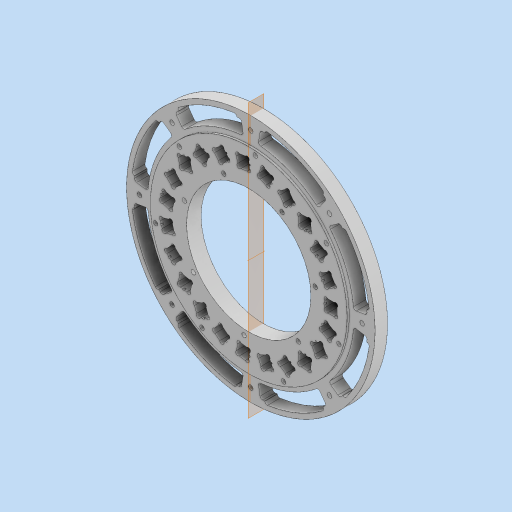
# Autodesk Inventor part: Ring_945
Saved by Autodesk Inventor 2024.2 (Build 282272000, 272)
## iProperties
Created: 2025-04-23
Part Number: Ring_945
Material: Generic
Document SubType Name: Modeling
Designer: 23661194
Density: 1 g/cm^3
Appearance: Default
Author: 23661194
Autodesk Inventor part; units mm, degrees
ref_plane "XZ Plane" through (0, 0, 0) normal (0, 1, 0) x (-1, 0, 0)
ref_plane "XY Plane" through (0, 0, 0) normal (0, 0, 1) x (1, 0, 0)
sketch "Shim Tray Slot_1" plane through (0, 0, 0) normal (0, 0, 1) x (1, 0, 0)
  line L0 (30.092, 109.0254) -> (29.9458, 108.3375)
  line L1 (33.5758, 105.3229) -> (31.6829, 97.1237)
  line L2 (-33.5758, 105.3229) -> (-31.6821, 97.1202)
  line L3 (-30.092, 109.0254) -> (-29.9458, 108.3375)
  arc A0 (-32.2001, 107.689) -> (-33.5758, 105.3229) centre (-31.6271, 105.7728) ccw
  arc A1 (29.147, 95.658) -> (-29.1504, 95.657) centre (0, 0) ccw
  arc A2 (28.6337, 111.3782) -> (-28.6337, 111.3782) centre (0, 0) ccw
  arc A3 (-29.9458, 108.3375) -> (-32.2001, 107.689) centre (0, 0) ccw
  arc A4 (32.2001, 107.689) -> (29.9458, 108.3375) centre (0, 0) ccw
  arc A5 (-28.6337, 111.3782) -> (-30.092, 109.0254) centre (-28.1357, 109.4412) ccw
  arc A6 (-31.6821, 97.1202) -> (-29.1504, 95.657) centre (-29.7334, 97.5701) ccw
  arc A7 (29.147, 95.658) -> (31.6829, 97.1237) centre (29.7309, 97.5743) ccw
  arc A8 (33.5758, 105.3229) -> (32.2001, 107.689) centre (31.6271, 105.7728) ccw
  arc A9 (30.092, 109.0254) -> (28.6337, 111.3782) centre (28.1357, 109.4412) ccw
  line L4 (0, 0) -> (0, 107.5)
  arc A10 (33.9656, 105.2329) -> (32.3146, 108.0722) centre (31.6271, 105.7728) ccw
  line L5 (33.9656, 105.2329) -> (32.0726, 97.0337)
  arc A11 (29.0304, 95.2754) -> (32.0726, 97.0337) centre (29.7309, 97.5743) ccw
  arc A12 (29.0304, 95.2754) -> (-29.0338, 95.2743) centre (0, 0) ccw
  arc A13 (-32.0718, 97.0302) -> (-29.0338, 95.2743) centre (-29.7334, 97.5701) ccw
  line L6 (-32.0718, 97.0302) -> (-33.9656, 105.2329)
  arc A14 (-32.3146, 108.0722) -> (-33.9656, 105.2329) centre (-31.6271, 105.7728) ccw
  arc A15 (-30.4152, 108.6221) -> (-32.3146, 108.0722) centre (0, 0) ccw
  line L7 (-30.4152, 108.6221) -> (-30.4833, 108.9422)
  arc A16 (-28.7333, 111.7656) -> (-30.4833, 108.9422) centre (-28.1357, 109.4412) ccw
  arc A17 (28.7333, 111.7656) -> (-28.7333, 111.7656) centre (0, 0) ccw
  arc A18 (30.4833, 108.9422) -> (28.7333, 111.7656) centre (28.1357, 109.4412) ccw
  line L8 (30.4833, 108.9422) -> (30.4152, 108.6221)
  arc A19 (32.3146, 108.0722) -> (30.4152, 108.6221) centre (0, 0) ccw
  dimension "d124" = 22.5
  dimension "d134" = 0.4
  measures "d134" radial gap between concentric circles of A2 A17
sketch "Shim Tray Slot_1_1" plane through (0, 0, 0) normal (0, 0, 1) x (1, 0, 0)
  line L0 (30.092, 109.0254) -> (29.9458, 108.3375)
  line L1 (33.5758, 105.3229) -> (31.6821, 97.1202)
  line L2 (-33.5758, 105.3229) -> (-31.6821, 97.1202)
  line L3 (-30.092, 109.0254) -> (-29.9458, 108.3375)
  arc A0 (-32.2001, 107.689) -> (-33.5758, 105.3229) centre (-31.6271, 105.7728) ccw
  arc A1 (29.1504, 95.657) -> (-29.1504, 95.657) centre (0, 0) ccw
  arc A2 (28.6337, 111.3782) -> (-28.6337, 111.3782) centre (0, 0) ccw
  arc A3 (-29.9458, 108.3375) -> (-32.2001, 107.689) centre (0, 0) ccw
  arc A4 (32.2001, 107.689) -> (29.9458, 108.3375) centre (0, 0) ccw
  arc A5 (-28.6337, 111.3782) -> (-30.092, 109.0254) centre (-28.1357, 109.4412) ccw
  arc A6 (-31.6821, 97.1202) -> (-29.1504, 95.657) centre (-29.7334, 97.5701) ccw
  arc A7 (29.1504, 95.657) -> (31.6821, 97.1202) centre (29.7309, 97.5743) ccw
  arc A8 (33.5758, 105.3229) -> (32.2001, 107.689) centre (31.6271, 105.7728) ccw
  arc A9 (30.092, 109.0254) -> (28.6337, 111.3782) centre (28.1357, 109.4412) ccw
  line L4 (0, 0) -> (0, 107.5)
  dimension "d125" = 22.5
  dimension "d126" = 22.5
sketch "Sketch1" plane through (0, 0, 0) normal (0, 0, 1) x (1, 0, 0)
  circle A0 centre (0, 0) radius 60
  circle A1 centre (0, 0) radius 120
  circle A2 centre (0, 0) radius 95
  dimension "d0" = 120
  dimension "d1" = 240
  dimension "d2" = 190
  constraints: 3 centre point, 3 coincident
  measures "d0" diameter of A0
  measures "d1" diameter of A1
  measures "d2" diameter of A2
extrude "Extrusion1" add sketch "Sketch1" along normal blind 12 contours A1 | A2
extrude "Extrusion2" add sketch "Sketch1" along normal blind 14 contours A2
sketch "Sketch3" plane through (0, 0, 14) normal (0, 0, 1) x (1, 0, 0)
  circle A0 centre (0, 0) radius 79.3546
  line L0 (79.3546, 0) -> (0, 0)
  line L1 (76.4119, 21.4096) -> (0, 0)
  line L2 (67.8021, 41.2314) -> (0, 0)
  line L3 (54.1637, 57.9952) -> (0, 0)
  line L4 (36.5083, 70.4577) -> (0, 0)
  line L5 (16.1452, 77.6948) -> (0, 0)
  line L6 (-5.4153, 79.1696) -> (0, 0)
  line L7 (-26.5742, 74.7727) -> (0, 0)
  line L8 (-45.7622, 64.8303) -> (0, 0)
  line L9 (-61.5562, 50.0797) -> (0, 0)
  line L10 (-72.7849, 31.6149) -> (0, 0)
  line L11 (-78.6155, 10.8054) -> (0, 0)
  line L12 (-78.6155, -10.8054) -> (0, 0)
  line L13 (-72.7849, -31.6149) -> (0, 0)
  line L14 (-61.5562, -50.0797) -> (0, 0)
  line L15 (-45.7622, -64.8303) -> (0, 0)
  line L16 (-26.5742, -74.7727) -> (0, 0)
  line L17 (-5.4153, -79.1696) -> (0, 0)
  line L18 (16.1452, -77.6948) -> (0, 0)
  line L19 (36.5083, -70.4577) -> (0, 0)
  line L20 (54.1637, -57.9952) -> (0, 0)
  line L21 (67.8021, -41.2314) -> (0, 0)
  line L22 (76.4119, -21.4096) -> (0, 0)
  line L23 (-168, 0) -> (168, 0) projected
  line L24 (85.2946, 5.94) -> (73.4146, 5.94)
  line L25 (73.4146, 5.94) -> (73.4146, -5.94)
  line L26 (73.4146, -5.94) -> (85.2946, -5.94)
  line L27 (85.2946, -5.94) -> (85.2946, 5.94)
  line L28 (85.2946, 5.94) -> (73.4146, -5.94) construction
  line L29 (73.4146, 5.94) -> (85.2946, -5.94) construction
  circle A1 centre (79.3546, 0) radius 2
  circle A2 centre (74.8276, -4.527) radius 2.1
  circle A3 centre (83.8816, -4.527) radius 2.1
  circle A4 centre (83.8816, 4.527) radius 2.1
  circle A5 centre (74.8276, 4.527) radius 2.1
  circle A6 centre (73.0546, 0) radius 0.75
  line L30 (73.0546, 0) -> (79.3546, 0)
  line L31 (78.4008, 29.5712) -> (68.2503, 23.3985)
  line L32 (68.2503, 23.3985) -> (74.423, 13.248)
  line L33 (74.423, 13.248) -> (84.5735, 19.4207)
  line L34 (84.5735, 19.4207) -> (78.4008, 29.5712)
  line L35 (78.4008, 29.5712) -> (74.423, 13.248) construction
  line L36 (68.2503, 23.3985) -> (84.5735, 19.4207) construction
  circle A7 centre (76.4119, 21.4096) radius 2
  circle A8 centre (74.8961, 15.1895) radius 2.1
  circle A9 centre (82.632, 19.8938) radius 2.1
  circle A10 centre (77.9277, 27.6297) radius 2.1
  circle A11 centre (70.1918, 22.9254) radius 2.1
  circle A12 centre (71.029, 18.1362) radius 0.75
  line L37 (71.029, 18.1362) -> (76.4119, 21.4096)
  line L38 (65.2608, 49.2382) -> (59.7953, 38.6901)
  line L39 (59.7953, 38.6901) -> (70.3433, 33.2245)
  line L40 (70.3433, 33.2245) -> (75.8089, 43.7726)
  line L41 (75.8089, 43.7726) -> (65.2608, 49.2382)
  line L42 (65.2608, 49.2382) -> (70.3433, 33.2245) construction
  line L43 (59.7953, 38.6901) -> (75.8089, 43.7726) construction
  circle A13 centre (67.8021, 41.2314) radius 2
  circle A14 centre (69.7388, 35.1292) radius 2.1
  circle A15 centre (73.9043, 43.1681) radius 2.1
  circle A16 centre (65.8653, 47.3335) radius 2.1
  circle A17 centre (61.6999, 39.2946) radius 2.1
  circle A18 centre (64.9037, 35.6377) radius 0.75
  line L44 (64.9037, 35.6377) -> (67.8021, 41.2314)
  line L45 (47.8322, 63.516) -> (48.6429, 51.6637)
  line L46 (48.6429, 51.6637) -> (60.4952, 52.4744)
  line L47 (60.4952, 52.4744) -> (59.6845, 64.3267)
  line L48 (59.6845, 64.3267) -> (47.8322, 63.516)
  line L49 (47.8322, 63.516) -> (60.4952, 52.4744) construction
  line L50 (48.6429, 51.6637) -> (59.6845, 64.3267) construction
  circle A19 centre (54.1637, 57.9952) radius 2
  circle A20 centre (58.9891, 53.7877) radius 2.1
  circle A21 centre (58.3712, 62.8206) radius 2.1
  circle A22 centre (49.3383, 62.2027) radius 2.1
  circle A23 centre (49.9562, 53.1698) radius 2.1
  circle A24 centre (54.5936, 51.7099) radius 0.75
  line L51 (54.5936, 51.7099) -> (54.1637, 57.9952)
  line L52 (28.23, 71.8851) -> (35.0809, 62.1795)
  line L53 (35.0809, 62.1795) -> (44.7865, 69.0304)
  line L54 (44.7865, 69.0304) -> (37.9356, 78.736)
  line L55 (37.9356, 78.736) -> (28.23, 71.8851)
  line L56 (28.23, 71.8851) -> (44.7865, 69.0304) construction
  line L57 (35.0809, 62.1795) -> (37.9356, 78.736) construction
  circle A25 centre (36.5083, 70.4577) radius 2
  circle A26 centre (42.8173, 69.37) radius 2.1
  circle A27 centre (37.5961, 76.7668) radius 2.1
  circle A28 centre (30.1992, 71.5455) radius 2.1
  circle A29 centre (35.4205, 64.1487) radius 2.1
  circle A30 centre (40.1413, 65.3108) radius 0.75
  line L58 (40.1413, 65.3108) -> (36.5083, 70.4577)
  line L59 (8.3304, 74.6131) -> (19.2269, 69.8801)
  line L60 (19.2269, 69.8801) -> (23.9599, 80.7765)
  line L61 (23.9599, 80.7765) -> (13.0634, 85.5095)
  line L62 (13.0634, 85.5095) -> (8.3304, 74.6131)
  line L63 (8.3304, 74.6131) -> (23.9599, 80.7765) construction
  line L64 (19.2269, 69.8801) -> (13.0634, 85.5095) construction
  circle A31 centre (16.1452, 77.6948) radius 2
  circle A32 centre (22.1009, 80.0434) radius 2.1
  circle A33 centre (13.7965, 83.6506) radius 2.1
  circle A34 centre (10.1894, 75.3461) radius 2.1
  circle A35 centre (18.4938, 71.739) radius 2.1
  circle A36 centre (21.9236, 75.1849) radius 0.75
  line L65 (21.9236, 75.1849) -> (16.1452, 77.6948)
  line L66 (-10.4912, 72.4761) -> (1.2782, 74.0937)
  line L67 (1.2782, 74.0937) -> (-0.3395, 85.8631)
  line L68 (-0.3395, 85.8631) -> (-12.1089, 84.2454)
  line L69 (-12.1089, 84.2454) -> (-10.4912, 72.4761)
  line L70 (-10.4912, 72.4761) -> (-0.3395, 85.8631) construction
  line L71 (1.2782, 74.0937) -> (-12.1089, 84.2454) construction
  circle A37 centre (-5.4153, 79.1696) radius 2
  circle A38 centre (-1.5469, 84.2708) radius 2.1
  circle A39 centre (-10.5166, 83.038) radius 2.1
  circle A40 centre (-9.2838, 74.0683) radius 2.1
  circle A41 centre (-0.3141, 75.3012) radius 2.1
  circle A42 centre (0.826, 80.0274) radius 0.75
  line L72 (0.826, 80.0274) -> (-5.4153, 79.1696)
  line L73 (-27.4333, 66.4163) -> (-18.2178, 73.9136)
  line L74 (-18.2178, 73.9136) -> (-25.7152, 83.1291)
  line L75 (-25.7152, 83.1291) -> (-34.9306, 75.6318)
  line L76 (-34.9306, 75.6318) -> (-27.4333, 66.4163)
  line L77 (-27.4333, 66.4163) -> (-25.7152, 83.1291) construction
  line L78 (-18.2178, 73.9136) -> (-34.9306, 75.6318) construction
  circle A43 centre (-26.5742, 74.7727) radius 2
  circle A44 centre (-25.9195, 81.1413) radius 2.1
  circle A45 centre (-32.9428, 75.4274) radius 2.1
  circle A46 centre (-27.2289, 68.4041) radius 2.1
  circle A47 centre (-20.2056, 74.118) radius 2.1
  circle A48 centre (-21.6872, 78.7486) radius 0.75
  line L79 (-21.6872, 78.7486) -> (-26.5742, 74.7727)
  line L80 (-42.1544, 57.2441) -> (-38.176, 68.4381)
  line L81 (-38.176, 68.4381) -> (-49.3701, 72.4165)
  line L82 (-49.3701, 72.4165) -> (-53.3484, 61.2224)
  line L83 (-53.3484, 61.2224) -> (-42.1544, 57.2441)
  line L84 (-42.1544, 57.2441) -> (-49.3701, 72.4165) construction
  line L85 (-38.176, 68.4381) -> (-53.3484, 61.2224) construction
  circle A49 centre (-45.7622, 64.8303) radius 2
  circle A50 centre (-48.5118, 70.6119) radius 2.1
  circle A51 centre (-51.5438, 62.0807) radius 2.1
  circle A52 centre (-43.0126, 59.0487) radius 2.1
  circle A53 centre (-39.9806, 67.5799) radius 2.1
  circle A54 centre (-43.6525, 70.7665) radius 0.75
  line L86 (-43.6525, 70.7665) -> (-45.7622, 64.8303)
  line L87 (-54.5319, 45.4725) -> (-56.949, 57.104)
  line L88 (-56.949, 57.104) -> (-68.5805, 54.6869)
  line L89 (-68.5805, 54.6869) -> (-66.1635, 43.0554)
  line L90 (-66.1635, 43.0554) -> (-54.5319, 45.4725)
  line L91 (-54.5319, 45.4725) -> (-68.5805, 54.6869) construction
  line L92 (-56.949, 57.104) -> (-66.1635, 43.0554) construction
  circle A55 centre (-61.5562, 50.0797) radius 2
  circle A56 centre (-66.9096, 53.591) radius 2.1
  circle A57 centre (-65.0675, 44.7264) radius 2.1
  circle A58 centre (-56.2029, 46.5684) radius 2.1
  circle A59 centre (-58.045, 55.4331) radius 2.1
  circle A60 centre (-62.838, 56.2479) radius 0.75
  line L93 (-62.838, 56.2479) -> (-61.5562, 50.0797)
  line L94 (-64.3894, 31.3281) -> (-72.4981, 40.0105)
  line L95 (-72.4981, 40.0105) -> (-81.1804, 31.9017)
  line L96 (-81.1804, 31.9017) -> (-73.0717, 23.2194)
  line L97 (-73.0717, 23.2194) -> (-64.3894, 31.3281)
  line L98 (-64.3894, 31.3281) -> (-81.1804, 31.9017) construction
  line L99 (-72.4981, 40.0105) -> (-73.0717, 23.2194) construction
  circle A61 centre (-72.7849, 31.6149) radius 2
  circle A62 centre (-79.1833, 31.8335) radius 2.1
  circle A63 centre (-73.0035, 25.2165) radius 2.1
  circle A64 centre (-66.3865, 31.3964) radius 2.1
  circle A65 centre (-72.5663, 38.0134) radius 2.1
  circle A66 centre (-77.085, 36.2192) radius 0.75
  line L100 (-77.085, 36.2192) -> (-72.7849, 31.6149)
  line L101 (-71.2931, 14.9226) -> (-82.7326, 18.1278)
  line L102 (-82.7326, 18.1278) -> (-85.9378, 6.6883)
  line L103 (-85.9378, 6.6883) -> (-74.4983, 3.4831)
  line L104 (-74.4983, 3.4831) -> (-71.2931, 14.9226)
  line L105 (-71.2931, 14.9226) -> (-85.9378, 6.6883) construction
  line L106 (-82.7326, 18.1278) -> (-74.4983, 3.4831) construction
  circle A67 centre (-78.6155, 10.8054) radius 2
  circle A68 centre (-84.1959, 7.6677) radius 2.1
  circle A69 centre (-75.4777, 5.2249) radius 2.1
  circle A70 centre (-73.035, 13.9432) radius 2.1
  circle A71 centre (-81.7532, 16.3859) radius 2.1
  circle A72 centre (-84.6818, 12.5052) radius 0.75
  line L107 (-84.6818, 12.5052) -> (-78.6155, 10.8054)
  line L108 (-74.4983, -3.4831) -> (-85.9378, -6.6883)
  line L109 (-85.9378, -6.6883) -> (-82.7326, -18.1278)
  line L110 (-82.7326, -18.1278) -> (-71.2931, -14.9226)
  line L111 (-71.2931, -14.9226) -> (-74.4983, -3.4831)
  line L112 (-74.4983, -3.4831) -> (-82.7326, -18.1278) construction
  line L113 (-85.9378, -6.6883) -> (-71.2931, -14.9226) construction
  circle A73 centre (-78.6155, -10.8054) radius 2
  circle A74 centre (-81.7532, -16.3859) radius 2.1
  circle A75 centre (-73.035, -13.9432) radius 2.1
  circle A76 centre (-75.4777, -5.2249) radius 2.1
  circle A77 centre (-84.1959, -7.6677) radius 2.1
  circle A78 centre (-84.6818, -12.5052) radius 0.75
  line L114 (-84.6818, -12.5052) -> (-78.6155, -10.8054)
  line L115 (-73.0717, -23.2194) -> (-81.1804, -31.9017)
  line L116 (-81.1804, -31.9017) -> (-72.4981, -40.0105)
  line L117 (-72.4981, -40.0105) -> (-64.3894, -31.3281)
  line L118 (-64.3894, -31.3281) -> (-73.0717, -23.2194)
  line L119 (-73.0717, -23.2194) -> (-72.4981, -40.0105) construction
  line L120 (-81.1804, -31.9017) -> (-64.3894, -31.3281) construction
  circle A79 centre (-72.7849, -31.6149) radius 2
  circle A80 centre (-72.5663, -38.0134) radius 2.1
  circle A81 centre (-66.3865, -31.3964) radius 2.1
  circle A82 centre (-73.0035, -25.2165) radius 2.1
  circle A83 centre (-79.1833, -31.8335) radius 2.1
  circle A84 centre (-77.085, -36.2192) radius 0.75
  line L121 (-77.085, -36.2192) -> (-72.7849, -31.6149)
  line L122 (-66.1635, -43.0554) -> (-68.5805, -54.6869)
  line L123 (-68.5805, -54.6869) -> (-56.949, -57.104)
  line L124 (-56.949, -57.104) -> (-54.5319, -45.4725)
  line L125 (-54.5319, -45.4725) -> (-66.1635, -43.0554)
  line L126 (-66.1635, -43.0554) -> (-56.949, -57.104) construction
  line L127 (-68.5805, -54.6869) -> (-54.5319, -45.4725) construction
  circle A85 centre (-61.5562, -50.0797) radius 2
  circle A86 centre (-58.045, -55.4331) radius 2.1
  circle A87 centre (-56.2029, -46.5684) radius 2.1
  circle A88 centre (-65.0675, -44.7264) radius 2.1
  circle A89 centre (-66.9096, -53.591) radius 2.1
  circle A90 centre (-62.838, -56.2479) radius 0.75
  line L128 (-62.838, -56.2479) -> (-61.5562, -50.0797)
  line L129 (-53.3484, -61.2224) -> (-49.3701, -72.4165)
  line L130 (-49.3701, -72.4165) -> (-38.176, -68.4381)
  line L131 (-38.176, -68.4381) -> (-42.1544, -57.2441)
  line L132 (-42.1544, -57.2441) -> (-53.3484, -61.2224)
  line L133 (-53.3484, -61.2224) -> (-38.176, -68.4381) construction
  line L134 (-49.3701, -72.4165) -> (-42.1544, -57.2441) construction
  circle A91 centre (-45.7622, -64.8303) radius 2
  circle A92 centre (-39.9806, -67.5799) radius 2.1
  circle A93 centre (-43.0126, -59.0487) radius 2.1
  circle A94 centre (-51.5438, -62.0807) radius 2.1
  circle A95 centre (-48.5118, -70.6119) radius 2.1
  circle A96 centre (-43.6525, -70.7665) radius 0.75
  line L135 (-43.6525, -70.7665) -> (-45.7622, -64.8303)
  line L136 (-34.9306, -75.6318) -> (-25.7152, -83.1291)
  line L137 (-25.7152, -83.1291) -> (-18.2178, -73.9136)
  line L138 (-18.2178, -73.9136) -> (-27.4333, -66.4163)
  line L139 (-27.4333, -66.4163) -> (-34.9306, -75.6318)
  line L140 (-34.9306, -75.6318) -> (-18.2178, -73.9136) construction
  line L141 (-25.7152, -83.1291) -> (-27.4333, -66.4163) construction
  circle A97 centre (-26.5742, -74.7727) radius 2
  circle A98 centre (-20.2056, -74.118) radius 2.1
  circle A99 centre (-27.2289, -68.4041) radius 2.1
  circle A100 centre (-32.9428, -75.4274) radius 2.1
  circle A101 centre (-25.9195, -81.1413) radius 2.1
  circle A102 centre (-21.6872, -78.7486) radius 0.75
  line L142 (-21.6872, -78.7486) -> (-26.5742, -74.7727)
  line L143 (-12.1089, -84.2454) -> (-0.3395, -85.8631)
  line L144 (-0.3395, -85.8631) -> (1.2782, -74.0937)
  line L145 (1.2782, -74.0937) -> (-10.4912, -72.4761)
  line L146 (-10.4912, -72.4761) -> (-12.1089, -84.2454)
  line L147 (-12.1089, -84.2454) -> (1.2782, -74.0937) construction
  line L148 (-0.3395, -85.8631) -> (-10.4912, -72.4761) construction
  circle A103 centre (-5.4153, -79.1696) radius 2
  circle A104 centre (-0.3141, -75.3012) radius 2.1
  circle A105 centre (-9.2838, -74.0683) radius 2.1
  circle A106 centre (-10.5166, -83.038) radius 2.1
  circle A107 centre (-1.5469, -84.2708) radius 2.1
  circle A108 centre (0.826, -80.0274) radius 0.75
  line L149 (0.826, -80.0274) -> (-5.4153, -79.1696)
  line L150 (13.0634, -85.5095) -> (23.9599, -80.7765)
  line L151 (23.9599, -80.7765) -> (19.2269, -69.8801)
  line L152 (19.2269, -69.8801) -> (8.3304, -74.6131)
  line L153 (8.3304, -74.6131) -> (13.0634, -85.5095)
  line L154 (13.0634, -85.5095) -> (19.2269, -69.8801) construction
  line L155 (23.9599, -80.7765) -> (8.3304, -74.6131) construction
  circle A109 centre (16.1452, -77.6948) radius 2
  circle A110 centre (18.4938, -71.739) radius 2.1
  circle A111 centre (10.1894, -75.3461) radius 2.1
  circle A112 centre (13.7965, -83.6506) radius 2.1
  circle A113 centre (22.1009, -80.0434) radius 2.1
  circle A114 centre (21.9236, -75.1849) radius 0.75
  line L156 (21.9236, -75.1849) -> (16.1452, -77.6948)
  line L157 (37.9356, -78.736) -> (44.7865, -69.0304)
  line L158 (44.7865, -69.0304) -> (35.0809, -62.1795)
  line L159 (35.0809, -62.1795) -> (28.23, -71.8851)
  line L160 (28.23, -71.8851) -> (37.9356, -78.736)
  line L161 (37.9356, -78.736) -> (35.0809, -62.1795) construction
  line L162 (44.7865, -69.0304) -> (28.23, -71.8851) construction
  circle A115 centre (36.5083, -70.4577) radius 2
  circle A116 centre (35.4205, -64.1487) radius 2.1
  circle A117 centre (30.1992, -71.5455) radius 2.1
  circle A118 centre (37.5961, -76.7668) radius 2.1
  circle A119 centre (42.8173, -69.37) radius 2.1
  circle A120 centre (40.1413, -65.3108) radius 0.75
  line L163 (40.1413, -65.3108) -> (36.5083, -70.4577)
  line L164 (59.6845, -64.3267) -> (60.4952, -52.4744)
  line L165 (60.4952, -52.4744) -> (48.6429, -51.6637)
  line L166 (48.6429, -51.6637) -> (47.8322, -63.516)
  line L167 (47.8322, -63.516) -> (59.6845, -64.3267)
  line L168 (59.6845, -64.3267) -> (48.6429, -51.6637) construction
  line L169 (60.4952, -52.4744) -> (47.8322, -63.516) construction
  circle A121 centre (54.1637, -57.9952) radius 2
  circle A122 centre (49.9562, -53.1698) radius 2.1
  circle A123 centre (49.3383, -62.2027) radius 2.1
  circle A124 centre (58.3712, -62.8206) radius 2.1
  circle A125 centre (58.9891, -53.7877) radius 2.1
  circle A126 centre (54.5936, -51.7099) radius 0.75
  line L170 (54.5936, -51.7099) -> (54.1637, -57.9952)
  line L171 (75.8089, -43.7726) -> (70.3433, -33.2245)
  line L172 (70.3433, -33.2245) -> (59.7953, -38.6901)
  line L173 (59.7953, -38.6901) -> (65.2608, -49.2382)
  line L174 (65.2608, -49.2382) -> (75.8089, -43.7726)
  line L175 (75.8089, -43.7726) -> (59.7953, -38.6901) construction
  line L176 (70.3433, -33.2245) -> (65.2608, -49.2382) construction
  circle A127 centre (67.8021, -41.2314) radius 2
  circle A128 centre (61.6999, -39.2946) radius 2.1
  circle A129 centre (65.8653, -47.3335) radius 2.1
  circle A130 centre (73.9043, -43.1681) radius 2.1
  circle A131 centre (69.7388, -35.1292) radius 2.1
  circle A132 centre (64.9037, -35.6377) radius 0.75
  line L177 (64.9037, -35.6377) -> (67.8021, -41.2314)
  line L178 (84.5735, -19.4207) -> (74.423, -13.248)
  line L179 (74.423, -13.248) -> (68.2503, -23.3985)
  line L180 (68.2503, -23.3985) -> (78.4008, -29.5712)
  line L181 (78.4008, -29.5712) -> (84.5735, -19.4207)
  line L182 (84.5735, -19.4207) -> (68.2503, -23.3985) construction
  line L183 (74.423, -13.248) -> (78.4008, -29.5712) construction
  circle A133 centre (76.4119, -21.4096) radius 2
  circle A134 centre (70.1918, -22.9254) radius 2.1
  circle A135 centre (77.9277, -27.6297) radius 2.1
  circle A136 centre (82.632, -19.8938) radius 2.1
  circle A137 centre (74.8961, -15.1895) radius 2.1
  circle A138 centre (71.029, -18.1362) radius 0.75
  line L184 (71.029, -18.1362) -> (76.4119, -21.4096)
  point P0 (75.8662, -28.0298)
  point P1 (79.9422, -27.0365)
  point P2 (83.0321, -21.9553)
  point P3 (82.0388, -17.8793)
  point P4 (76.9576, -14.7894)
  point P5 (72.8816, -15.7827)
  point P6 (69.7917, -20.8639)
  point P7 (70.785, -24.9399)
  point P8 (61.16, -41.324)
  point P9 (63.896, -46.6043)
  point P10 (67.8948, -47.8734)
  point P11 (73.175, -45.1374)
  point P12 (74.4441, -41.1387)
  point P13 (71.7081, -35.8585)
  point P14 (67.7094, -34.5893)
  point P15 (62.4292, -37.3253)
  point P16 (60.2928, -55.434)
  point P17 (57.5356, -52.2719)
  point P18 (51.6025, -51.8661)
  point P19 (48.4405, -54.6233)
  point P20 (48.0346, -60.5564)
  point P21 (50.7918, -63.7184)
  point P22 (56.7249, -64.1242)
  point P23 (59.8869, -61.3671)
  point P24 (29.9407, -69.4615)
  point P25 (30.6535, -73.5958)
  point P26 (35.512, -77.0253)
  point P27 (39.6463, -76.3125)
  point P28 (43.0758, -71.454)
  point P29 (42.363, -67.3197)
  point P30 (37.5045, -63.8902)
  point P31 (33.3702, -64.603)
  point P32 (11.8816, -82.7886)
  point P33 (15.7844, -84.3277)
  point P34 (21.239, -81.9584)
  point P35 (22.778, -78.0556)
  point P36 (20.4088, -72.601)
  point P37 (16.506, -71.0619)
  point P38 (11.0514, -73.4312)
  point P39 (9.5123, -77.334)
  point P40 (0.8742, -77.0326)
  point P41 (-1.6607, -73.6898)
  point P42 (-7.5523, -72.88)
  point P43 (-10.8951, -75.415)
  point P44 (-11.7049, -81.3065)
  point P45 (-9.17, -84.6494)
  point P46 (-3.2784, -85.4591)
  point P47 (0.0644, -82.9242)
  point P48 (-25.1321, -68.2885)
  point P49 (-29.3054, -68.7175)
  point P50 (-33.0585, -73.3306)
  point P51 (-32.6294, -77.5039)
  point P52 (-28.0163, -81.257)
  point P53 (-23.843, -80.8279)
  point P54 (-20.09, -76.2148)
  point P55 (-20.519, -72.0415)
  point P56 (-52.355, -64.0177)
  point P57 (-50.3635, -69.6213)
  point P58 (-46.5748, -71.4231)
  point P59 (-40.9712, -69.4316)
  point P60 (-39.1694, -65.6429)
  point P61 (-41.1609, -60.0393)
  point P62 (-44.9496, -58.2375)
  point P63 (-50.5532, -60.229)
  point P64 (-56.3454, -54.1995)
  point P65 (-55.1355, -48.377)
  point P66 (-57.4364, -44.8689)
  point P67 (-63.259, -43.659)
  point P68 (-66.767, -45.9599)
  point P69 (-67.977, -51.7825)
  point P70 (-65.676, -55.2905)
  point P71 (-59.8535, -56.5004)
  point P72 (-70.9037, -25.2442)
  point P73 (-75.0965, -25.3875)
  point P74 (-79.1556, -29.7337)
  point P75 (-79.0124, -33.9266)
  point P76 (-74.6661, -37.9857)
  point P77 (-70.4733, -37.8424)
  point P78 (-66.4142, -33.4962)
  point P79 (-66.5574, -29.3033)
  point P80 (-73.698, -6.3396)
  point P81 (-77.3548, -4.2835)
  point P82 (-83.0813, -5.888)
  point P83 (-85.1374, -9.5448)
  point P84 (-83.5329, -15.2713)
  point P85 (-79.8761, -17.3274)
  point P86 (-74.1496, -15.7229)
  point P87 (-72.0935, -12.0661)
  point P88 (-72.0935, 12.0661)
  point P89 (-74.1496, 15.7229)
  point P90 (-79.8761, 17.3274)
  point P91 (-83.5329, 15.2713)
  point P92 (-85.1374, 9.5448)
  point P93 (-83.0813, 5.888)
  point P94 (-77.3548, 4.2835)
  point P95 (-73.698, 6.3396)
  point P96 (-66.5574, 29.3033)
  point P97 (-66.4142, 33.4962)
  point P98 (-70.4733, 37.8424)
  point P99 (-74.6661, 37.9857)
  point P100 (-79.0124, 33.9266)
  point P101 (-79.1556, 29.7337)
  point P102 (-75.0965, 25.3875)
  point P103 (-70.9037, 25.2442)
  point P104 (-57.4364, 44.8689)
  point P105 (-55.1355, 48.377)
  point P106 (-56.3454, 54.1995)
  point P107 (-59.8535, 56.5004)
  point P108 (-65.676, 55.2905)
  point P109 (-67.977, 51.7825)
  point P110 (-66.767, 45.9599)
  point P111 (-63.259, 43.659)
  point P112 (-44.9496, 58.2375)
  point P113 (-41.1609, 60.0393)
  point P114 (-39.1694, 65.6429)
  point P115 (-40.9712, 69.4316)
  point P116 (-46.5748, 71.4231)
  point P117 (-50.3635, 69.6213)
  point P118 (-52.355, 64.0177)
  point P119 (-50.5532, 60.229)
  point P120 (-20.519, 72.0415)
  point P121 (-20.09, 76.2148)
  point P122 (-23.843, 80.8279)
  point P123 (-28.0163, 81.257)
  point P124 (-32.6294, 77.5039)
  point P125 (-33.0585, 73.3306)
  point P126 (-29.3054, 68.7175)
  point P127 (-25.1321, 68.2885)
  point P128 (-10.8951, 75.415)
  point P129 (-7.5523, 72.88)
  point P130 (-1.6607, 73.6898)
  point P131 (0.8742, 77.0326)
  point P132 (0.0644, 82.9242)
  point P133 (-3.2784, 85.4591)
  point P134 (-9.17, 84.6494)
  point P135 (-11.7049, 81.3065)
  point P136 (9.5123, 77.334)
  point P137 (11.0514, 73.4312)
  point P138 (16.506, 71.0619)
  point P139 (20.4088, 72.601)
  point P140 (22.778, 78.0556)
  point P141 (21.239, 81.9584)
  point P142 (15.7844, 84.3277)
  point P143 (11.8816, 82.7886)
  point P144 (29.9407, 69.4615)
  point P145 (33.3702, 64.603)
  point P146 (37.5045, 63.8902)
  point P147 (42.363, 67.3197)
  point P148 (43.0758, 71.454)
  point P149 (39.6463, 76.3125)
  point P150 (35.512, 77.0253)
  point P151 (30.6535, 73.5958)
  point P152 (60.2928, 55.434)
  point P153 (59.8869, 61.3671)
  point P154 (56.7249, 64.1242)
  point P155 (50.7918, 63.7184)
  point P156 (48.0346, 60.5564)
  point P157 (48.4405, 54.6233)
  point P158 (51.6025, 51.8661)
  point P159 (57.5356, 52.2719)
  point P160 (71.7081, 35.8585)
  point P161 (74.4441, 41.1387)
  point P162 (73.175, 45.1374)
  point P163 (67.8948, 47.8734)
  point P164 (63.896, 46.6043)
  point P165 (61.16, 41.324)
  point P166 (62.4292, 37.3253)
  point P167 (67.7094, 34.5893)
  point P168 (70.785, 24.9399)
  point P169 (69.7917, 20.8639)
  point P170 (72.8816, 15.7827)
  point P171 (76.9576, 14.7894)
  point P172 (82.0388, 17.8793)
  point P173 (83.0321, 21.9553)
  point P174 (79.9422, 27.0365)
  point P175 (75.8662, 28.0298)
  point P176 (76.3811, 5.94)
  point P177 (73.4146, 2.9735)
  point P178 (73.4146, -2.9735)
  point P179 (76.3811, -5.94)
  point P180 (82.328, -5.94)
  point P181 (85.2946, -2.9735)
  point P182 (85.2946, 2.9735)
  point P183 (82.328, 5.94)
  dimension "d65" = 158.7091
  dimension "d71" = -31.304
  dimension "d72" = -62.609
  dimension "d73" = -93.913
  dimension "d74" = -125.217
  dimension "d75" = -156.522
  dimension "d76" = -187.826
  dimension "d77" = -219.13
  dimension "d78" = -250.435
  dimension "d79" = -281.739
  dimension "d80" = -313.043
  dimension "d81" = -344.348
  dimension "d82" = -15.652
  dimension "d83" = -46.957
  dimension "d84" = -78.261
  dimension "d85" = -109.565
  dimension "d86" = -140.87
  dimension "d87" = -172.174
  dimension "d88" = -203.478
  dimension "d89" = 3.6331
  dimension "d90" = -234.783
  dimension "d91" = -266.087
  dimension "d92" = -297.391
  dimension "d93" = -328.696
  dimension "d68" = 360
  dimension "d70" = 0
  constraints: 46 end point, 1 coincident, 1 horizontal, 1 horizontal alignment, 96 other
  measures "d70" vertical extent of L0
extrude "Extrusion3" cut sketch "Sketch3" against normal blind 12 contours L0 A1 A0 | L23 A1 A0 | A0 A1 L0 | A0 A1 L23 | A1 L0 A6 L25 A5 L24 A0 | A0 L24 A4 L27 L23 A1 | A1 L23 L27 A3 L26 A0 | A0 L26 A2 L25 A6 L0 A1 | A6 L25 L0 | L0 L25 A6 | L33 A8 L32 A12 L37 A7 A0 | A0 A7 L31 A10 L34 A9 L33 | A4 L27 L24 | L24 L27 A4 | A5 L25 L24 | L24 L25 A5 | L178 A136 L181 A135 L180 A0 A133 | A0 A133 L184 A138 L179 A137 L178 | A2 L25 L26 | L26 L25 A2 | A3 L27 L26 | L26 L27 A3 | A7 L37 A0 | A0 A7 | A8 L32 L33 | L33 L32 A8 | A9 L34 L33 | L33 L34 A9 | A133 A0 | A0 L184 A133 | A136 L181 L178 | L178 L181 A136 | A137 L179 L178 | L178 L179 A137 | L1 A7 A0 | L37 A7 L1 | L37 A12 L32 L1 A7 | A0 A133 L22 | L22 A133 L184 | A133 L22 L179 A138 L184 | A7 L1 L32 A11 L31 A0 | L37 L32 A12 | A12 L32 L37 | A10 L31 L34 | L34 L31 A10 | A0 L180 A134 L179 L22 A133 | L184 L179 A138 | A138 L179 L184 | A135 L180 L181 | L181 L180 A135 | A17 L38 L39 L2 | L2 L39 A17 | A23 L45 L3 | L3 L45 L46 A23 | A29 L52 L4 | L4 L52 L53 A29 | L59 A34 L62 A0 A31 L5 | L5 A31 L65 A36 L60 A35 L59 | L66 A40 L69 A0 A37 L6 | L6 A37 A0 A42 L67 A41 L66 | L73 A46 L76 A0 A43 L7 | L7 A43 A0 L74 A47 L73 | A52 L83 L80 L8 | L8 L80 A52 | A58 L90 L9 | L9 L90 L87 A58 | L97 A63 L96 A0 A61 L10 | L10 A61 A0 L94 A64 L97 | L104 A69 L103 A0 A67 L11 | L11 A67 A0 L101 A70 L104 | L111 A75 L110 A0 A73 L12 | L12 A73 A0 L108 A76 L111 | L118 A81 L117 A0 A79 L13 | L13 A79 A0 L115 A82 L118 | A87 L124 L125 L14 | L14 L125 A87 | A93 L131 L15 | L15 L131 L132 A93 | L138 A98 L137 A0 A97 L16 | L16 A97 A0 L139 A99 L138 | L145 A104 L144 A108 A0 A103 L17 | L17 A103 A0 L146 A105 L145 | L152 A110 L151 A114 L156 A109 L18 | L18 A109 A0 L153 A111 L152 | A116 L158 L159 L19 | L19 L159 A116 | A122 L165 L166 L20 | L20 L166 A122 | A128 L172 L21 | L21 L172 L173 A128 | A11 L31 L32 | L32 L31 A11 | L39 L38 A17 L2 | L2 A17 L39 | L38 A16 A0 A13 L2 A17 | A17 L2 A13 L44 A18 L39 | L45 A23 L3 | L3 A23 L46 L45 | L45 A22 A0 A19 L3 A23 | A23 L3 A19 L51 A24 L46 | L52 A29 L4 | L4 A29 L53 L52 | L52 A28 A0 A25 L4 A29 | A29 L4 A25 L58 A30 L53 | A31 A0 L5 | L5 L65 A31 | A34 L62 L59 | L59 L62 A34 | A35 L60 L59 | L59 L60 A35 | A37 A0 L6 | L6 A0 A37 | A40 L69 L66 | L66 L69 A40 | A41 L67 L66 | L66 L67 A41 | A43 A0 L7 | L7 A0 A43 | A46 L76 L73 | L73 L76 A46 | A47 L74 L73 | L73 L74 A47 | L80 L83 A52 L8 | L8 A52 L80 | L83 A51 A0 A49 L8 A52 | L90 A58 L9 | L9 A58 L87 L90 | L90 A57 A0 A55 L9 A58 | A61 A0 L10 | L10 A0 A61 | A63 L96 L97 | L97 L96 A63 | A64 L94 L97 | L97 L94 A64 | A67 A0 L11 | L11 A0 A67 | A69 L103 L104 | L104 L103 A69 | A70 L101 L104 | L104 L101 A70 | A73 A0 L12 | L12 A0 A73 | A75 L110 L111 | L111 L110 A75 | A76 L108 L111 | L111 L108 A76 | A79 A0 L13 | L13 A0 A79 | A81 L117 L118 | L118 L117 A81 | A82 L115 L118 | L118 L115 A82 | L125 L124 A87 L14 | L14 A87 L125 | A87 L14 A85 A0 A88 L125 | L131 A93 L15 | L15 A93 L132 L131 | A93 L15 A91 A0 A94 L132 | A97 A0 L16 | L16 A0 A97 | A98 L137 L138 | L138 L137 A98 | A99 L139 L138 | L138 L139 A99 | A103 A0 L17 | L17 A0 A103 | A104 L144 L145 | L145 L144 A104 | A105 L146 L145 | L145 L146 A105 | A109 L156 L18 | L18 A0 A109 | A110 L151 L152 | L152 L151 A110 | A111 L153 L152 | L152 L153 A111 | L159 L158 A116 L19 | L19 A116 L159 | L158 A120 L163 A115 L19 A116 | A116 L19 A115 A0 A117 L159 | L166 L165 A122 L20 | L20 A122 L166 | L165 A126 L170 A121 L20 A122 | A122 L20 A121 A0 A123 L166 | L172 A128 L21 | L21 A128 L173 L172 | L172 A132 L177 A127 L21 A128 | A128 L21 A127 A0 A129 L173 | A134 L180 L179 | L179 L180 A134 | L103 A68 L102 A72 L107 A67 A0 | A0 A73 L114 A78 L109 A77 L108 | A14 L39 L40 A0 | A0 L40 A14 | A131 L171 A0 | A0 L171 L172 A131 | A16 A0 L38 | L38 A0 A16 | A18 L44 L39 | A22 A0 L45 | L45 A0 A22 | A24 L51 L46 | A28 A0 L55 L52 | L52 L55 A0 A28 | A30 L58 L53 | A0 A31 | A0 A31 L65 | A0 L62 A33 L61 A32 L60 A31 | A31 A0 L60 A36 L65 | L72 A37 A0 | A0 A37 L72 | A0 L69 A39 L68 A38 L67 A42 L72 A37 | L79 A43 A0 | A0 A43 L79 | A0 L76 A45 L75 A44 L74 A48 L79 A43 | L8 A49 A0 A53 L80 A52 | A51 A0 L83 | L83 A0 A51 | L9 A55 A0 A59 L87 A58 | A57 A0 L89 L90 | L90 L89 A0 A57 | L100 A61 A0 | A0 A61 L100 | A0 L96 A62 L95 A66 L100 A61 | L107 A67 A0 | A0 A67 L107 | L114 A73 A0 | A0 A73 L114 | L121 A79 A0 | A0 A79 L121 | A79 L121 A84 L116 A83 L115 A0 | A87 L124 A86 A0 A85 L14 | A88 A0 L122 L125 | L125 L122 A0 A88 | A93 L131 A92 A0 A91 L15 | A94 A0 L132 | L132 A0 A94 | L142 A97 A0 | A0 A97 L142 | A97 L142 A102 L137 A101 L136 A100 L139 A0 | L149 A103 A0 | A0 A103 L149 | A103 L149 A108 L144 A107 L143 A106 L146 A0 | A0 A109 | L156 A109 A0 | L156 A114 L151 A0 A109 | A109 A0 L151 A113 L150 A112 L153 | L158 L163 A120 | A117 A0 L160 L159 | L159 L160 A0 A117 | L165 L170 A126 | A123 A0 L166 | L166 A0 A123 | L172 L177 A132 | A129 A0 L173 | L173 A0 A129 | A68 L102 L103 | L103 L102 A68 | A77 L109 L108 | L108 L109 A77 | L40 L39 A14 A0 | A0 A14 L40 | L39 A18 L44 A13 A0 A14 | L171 A131 A0 | A0 A131 L172 L171 | A131 A0 A127 L177 A132 L172 | A13 A0 L2 | L2 L44 A13 | L38 L41 A16 A0 | A0 A16 L41 L38 | A16 L41 A15 L40 A14 A0 A13 | L44 A18 L39 | A19 A0 L3 | L3 L51 A19 | L45 L48 A22 A0 | A0 A22 L48 L45 | A22 L48 A21 L47 A20 A0 A19 | L51 A24 L46 | L51 A19 A0 A20 L46 A24 | A25 A0 L4 | L4 L58 A25 | A28 L55 A0 | L58 A30 L53 | L58 A25 A0 L53 A30 | L65 L60 A36 | A36 L60 L65 | A37 L72 A42 A0 | A42 A0 L67 | A43 L79 A48 L74 A0 | A49 A0 L8 | L8 A0 A49 | A53 A0 L81 L80 | L80 L81 A0 A53 | L83 L82 A51 A0 | A0 A51 L82 L83 | A51 L82 A50 L81 A54 L86 A49 A0 | A55 A0 L9 | L9 A0 A55 | A57 L89 A0 | A59 A0 L87 | L87 A0 A59 | A61 L100 A66 L95 A65 L94 A0 | A67 L107 A72 L102 A71 L101 A0 | A0 L110 A74 L109 A78 L114 A73 | A0 L117 A80 L116 A84 L121 A79 | A85 A0 L14 | L14 A0 A85 | A86 A0 L124 | L124 A0 A86 | A0 L122 A88 | A91 A0 L15 | L15 A0 A91 | A92 A0 L130 L131 | L131 L130 A0 A92 | L132 L129 A94 A0 | A0 A94 L129 L132 | A0 A91 L135 A96 L130 A95 L129 A94 | A0 L137 A102 L142 A97 | A0 A108 L149 A103 | L144 A0 A108 | L156 L151 A114 | A114 L151 L156 | A115 L163 L19 | L19 A0 A115 | L158 A120 L163 | A120 L158 A0 A115 L163 | A0 L160 A117 | A121 L170 L20 | L20 A0 A121 | L165 A126 L170 | A126 L165 A125 A0 A121 L170 | L166 L167 A123 A0 | A0 A123 L167 L166 | A0 A121 A125 L164 A124 L167 A123 | A127 L177 L21 | L21 A0 A127 | L172 A132 L177 | L173 L174 A129 A0 | A0 A129 L174 L173 | A0 A127 A131 L171 A130 L174 A129 | A0 A13 | A0 A13 L44 | A20 L46 A0 | A0 L46 L47 A20 | A0 A19 | A0 A19 L51 | A0 A25 A28 L55 A27 L54 A26 L53 | A0 A25 | A0 A25 L58 | L55 A28 A0 | A33 L61 L62 | L62 L61 A33 | A42 L72 L67 A0 | A42 L67 L72 | A39 L68 L69 | L69 L68 A39 | L79 L74 A48 | A48 L74 L79 | A0 L81 A53 | A45 L75 L76 | L76 L75 A45 | L86 A49 A0 | A0 A49 L86 | A53 L81 A0 | A0 A49 L86 A54 L81 A53 | A0 L87 L88 A59 | L93 A55 A0 | A0 A55 L93 | A0 A57 L89 A56 L88 A60 L93 A55 | L89 A57 A0 | A0 A59 L88 L87 | A0 A55 L93 A60 L88 A59 | L100 L95 A66 | A66 L95 L100 | A62 L95 L96 | L96 L95 A62 | A65 L95 L94 | L94 L95 A65 | L107 L102 A72 | A72 L102 L107 | A71 L102 L101 | L101 L102 A71 | L114 L109 A78 | A78 L109 L114 | A74 L109 L110 | L110 L109 A74 | L121 L116 A84 | A84 L116 L121 | A83 L116 L115 | L115 L116 A83 | A80 L116 L117 | L117 L116 A80 | L128 A85 A0 | A0 A85 L128 | A85 L128 A90 L123 A89 L122 A88 A0 | L124 L123 A86 A0 | A0 A86 L123 L124 | A86 L123 A90 L128 A85 A0 | A0 A88 L122 | L135 A91 A0 | A0 A91 L135 | A92 L130 A96 L135 A91 A0 | A0 L130 A92 | L142 L137 A102 | A102 L137 L142 | A92 L130 A0 | A100 L136 L139 | L139 L136 A100 | A0 L144 L149 A108 | L149 L144 A108 | A106 L143 L146 | L146 L143 A106 | A112 L150 L153 | L153 L150 A112 | A0 A115 | L163 A115 A0 | A115 A0 L158 A119 L157 A118 L160 A117 | A0 A117 L160 | A0 A121 | L170 A121 A0 | A0 A127 | L177 A127 A0 | A125 L164 L165 A0 | A0 L165 A125 | A15 L41 L40 | L40 L41 A15 | A130 L174 L171 | L171 L174 A130 | L46 A20 A0 | A0 A20 L47 L46 | A26 L54 L53 | L53 L54 A26 | A21 L47 L48 | L48 L47 A21 | A32 L61 L60 | L60 L61 A32 | A27 L54 L55 | L55 L54 A27 | A50 L81 L82 | L82 L81 A50 | A56 L88 L89 | L89 L88 A56 | A89 L123 L122 | L122 L123 A89 | A95 L130 L129 | L129 L130 A95 | A113 L150 L151 | L151 L150 A113 | A118 L157 L160 | L160 L157 A118 | L165 A0 A125 | A119 L157 L158 | L158 L157 A119 | A124 L164 L167 | L167 L164 A124 | L165 L164 A125 A0 | A38 L68 L67 | L67 L68 A38 | A44 L75 L74 | L74 L75 A44 | A54 L86 L81 | A54 L81 L86 | A60 L93 L88 | A60 L88 L93 | L128 L123 A90 | A90 L123 L128 | L135 L130 A96 | A96 L130 L135 | A101 L136 L137 | L137 L136 A101 | A107 L143 L144 | L144 L143 A107 picked at (73.4584, -0.4081) picked at (73.4584, 0.4081) picked at (0.5509, 79.338) picked at (0.5509, -79.338)
extrude "Extrusion4" cut sketch "Sketch3" against normal blind 2 contours A6 L25 L0 | L0 L25 A6 | L25 A6 L0 | L0 A6 L25 | L37 L32 A12 | A12 L32 L37 | A12 L32 | L184 L179 A138 | A138 L179 L184 | L179 A138 | A18 L44 L39 | L39 A18 | A24 L51 L46 | L46 A24 | A30 L58 L53 | L53 A30 | A120 L158 | L158 L163 A120 | A126 L165 | L165 L170 A126 | A132 L172 | L172 L177 A132 | L44 A18 L39 | L51 A24 L46 | L58 A30 L53 | L65 L60 A36 | A36 L60 L65 | L60 A36 | A42 A0 L67 | L67 A0 A42 | A108 A0 L144 | L144 A0 A108 | L156 L151 A114 | A114 L151 L156 | A114 L151 | L158 A120 L163 | L165 A126 L170 | L172 A132 L177 | A0 L67 A42 | A42 L72 L67 A0 | A42 L67 L72 | L79 L74 A48 | A48 L74 L79 | L74 A48 | L100 L95 A66 | A66 L95 L100 | L107 L102 A72 | A72 L102 L107 | L114 L109 A78 | A78 L109 L114 | L121 L116 A84 | A84 L116 L121 | L142 L137 A102 | A102 L137 L142 | A102 L137 | A0 L144 L149 A108 | L149 L144 A108 | A0 A108 L144 | A72 L102 | L109 A78 | A66 L95 | L116 A84 | A54 L86 L81 | L81 A54 | A54 L81 L86 | A60 L93 L88 | L88 A60 | A60 L88 L93 | L128 L123 A90 | A90 L123 L128 | A90 L123 | L135 L130 A96 | A96 L130 L135 | A96 L130
extrude "Extrusion5" cut sketch "Sketch3" against normal through all contours L0 A1 A0 | L23 A1 A0 | A0 A1 L0 | A0 A1 L23 | A7 L37 A0 | A0 A7 | A133 A0 | A0 L184 A133 | L1 A7 A0 | L37 A7 L1 | A0 A133 L22 | L22 A133 L184 | A31 A0 L5 | L5 L65 A31 | A37 A0 L6 | L6 A0 A37 | A43 A0 L7 | L7 A0 A43 | A61 A0 L10 | L10 A0 A61 | A67 A0 L11 | L11 A0 A67 | A73 A0 L12 | L12 A0 A73 | A79 A0 L13 | L13 A0 A79 | A97 A0 L16 | L16 A0 A97 | A103 A0 L17 | L17 A0 A103 | A109 L156 L18 | L18 A0 A109 | A0 A31 | A0 A31 L65 | L72 A37 A0 | A0 A37 L72 | L79 A43 A0 | A0 A43 L79 | L100 A61 A0 | A0 A61 L100 | L107 A67 A0 | A0 A67 L107 | L114 A73 A0 | A0 A73 L114 | L121 A79 A0 | A0 A79 L121 | L142 A97 A0 | A0 A97 L142 | L149 A103 A0 | A0 A103 L149 | A0 A109 | L156 A109 A0 | A13 A0 L2 | L2 L44 A13 | A19 A0 L3 | L3 L51 A19 | A25 A0 L4 | L4 L58 A25 | A49 A0 L8 | L8 A0 A49 | A55 A0 L9 | L9 A0 A55 | A85 A0 L14 | L14 A0 A85 | A91 A0 L15 | L15 A0 A91 | A115 L163 L19 | L19 A0 A115 | A121 L170 L20 | L20 A0 A121 | A127 L177 L21 | L21 A0 A127 | A0 A13 | A0 A13 L44 | A0 A19 | A0 A19 L51 | A0 A25 | A0 A25 L58 | L86 A49 A0 | A0 A49 L86 | L93 A55 A0 | A0 A55 L93 | L128 A85 A0 | A0 A85 L128 | L135 A91 A0 | A0 A91 L135 | A0 A115 | L163 A115 A0 | A0 A121 | L170 A121 A0 | A0 A127 | L177 A127 A0
sketch "Sketch4" plane through (0, 0, 12) normal (0, 0, 1) x (1, 0, 0)
  circle A0 centre (0, 0) radius 107.5
  circle A1 centre (0, 107.5) radius 2.15
  circle A2 centre (-76.014, 76.014) radius 2.15
  circle A3 centre (-107.5, 0) radius 2.15
  circle A4 centre (-76.014, -76.014) radius 2.15
  circle A5 centre (0, -107.5) radius 2.15
  circle A6 centre (76.014, -76.014) radius 2.15
  circle A7 centre (107.5, 0) radius 2.15
  circle A8 centre (76.014, 76.014) radius 2.15
  dimension "d100" = 215
  dimension "d101" = 4.3
  dimension "d104" = 360
  constraints: 8 centre point, 1 coincident, 1 vertical alignment, 19 other
  measures "d101" diameter of A1
extrude "Extrusion6" cut sketch "Sketch4" against normal through all contours A0 A7 | A0 A7 | A8 A0 | A0 A8 | A6 A0 | A0 A6 | A1 A0 | A0 A1 | A5 A0 | A0 A5 | A2 A0 | A0 A2 | A4 A0 | A0 A4 | A3 A0 | A0 A3
sketch "Sketch5" plane through (0, 0, 14) normal (0, 0, 1) x (1, 0, 0)
  circle A0 centre (0, 0) radius 91
  circle A1 centre (0, 0) radius 65
  circle A2 centre (0, 0) radius 60 projected
  line L0 (0, 0) -> (6.3478, 90.7783)
  line L1 (0, 168) -> (0, -168) projected
  circle A3 centre (6.3478, 90.7783) radius 2.1
  circle A4 centre (-67.0155, 61.5623) radius 2.1
  circle A5 centre (-89.9149, -14.0114) radius 2.1
  circle A6 centre (-45.1064, -79.0342) radius 2.1
  circle A7 centre (33.668, -84.5427) radius 2.1
  circle A8 centre (87.0898, -26.3888) radius 2.1
  circle A9 centre (74.9312, 51.6364) radius 2.1
  line L2 (0, 0) -> (32.2189, 56.453)
  circle A10 centre (32.2189, 56.453) radius 2.1
  circle A11 centre (-24.0486, 60.3876) radius 2.1
  circle A12 centre (-62.207, 18.8491) radius 2.1
  circle A13 centre (-53.5223, -36.8832) radius 2.1
  circle A14 centre (-4.5342, -64.8417) radius 2.1
  circle A15 centre (47.8682, -43.9731) radius 2.1
  circle A16 centre (64.2249, 10.0081) radius 2.1
  dimension "d108" = 182
  dimension "d109" = 130
  dimension "d110" = 4
  dimension "d111" = 4.2
  dimension "d114" = 360
  dimension "d116" = 29.714
  dimension "d117" = 4.2
  dimension "d120" = 360
  constraints: 14 centre point, 4 coincident, 4 end point, 36 other
  measures "d110" angle of L1 L0
  measures "d111" diameter of A3
  measures "d116" angle of L1 L2
  measures "d117" diameter of A10
extrude "Extrusion7" cut sketch "Sketch5" against normal blind 8 contours A9 A0 | A0 A9 | A8 A0 | A0 A8 | A3 L0 A0 | A0 A3 | A7 A0 | A0 A7 | L0 A3 A0 | A10 A1 | A1 L2 A10 | A6 A0 | A0 A6 | A4 A0 | A0 A4 | A1 A10 L2 | A11 A1 | A1 A11 | A14 A1 | A1 A14 | A15 A1 | A1 A15 | A5 A0 | A0 A5 | A16 A1 | A1 A16 | A12 A1 | A1 A12 | A13 A1 | A1 A13
sketch "Sketch6" plane through (0, 0, 12) normal (0, 0, 1) x (1, 0, 0)
  line L0 (0, 168) -> (0, -168) projected
  line L1 (69.5236, 89.2106) -> (69.1253, 88.631)
  line L2 (71.3254, 84.4568) -> (66.4388, 77.6061)
  line L3 (9.2853, 110.1546) -> (7.8959, 101.8516)
  line L4 (13.9208, 112.2421) -> (13.7927, 111.5505)
  arc A0 (11.4618, 111.8141) -> (9.2853, 110.1546) centre (11.2579, 109.8245) ccw
  arc A1 (63.5351, 77.2224) -> (9.6749, 99.5309) centre (0, 0) ccw
  arc A2 (69.0767, 91.9424) -> (16.1685, 113.8577) centre (0, 0) ccw
  arc A3 (13.7927, 111.5505) -> (11.4618, 111.8141) centre (0, 0) ccw
  arc A4 (70.9598, 87.1692) -> (69.1253, 88.631) centre (0, 0) ccw
  arc A5 (16.1685, 113.8577) -> (13.9208, 112.2421) centre (15.8873, 111.8776) ccw
  arc A6 (7.8959, 101.8516) -> (9.6749, 99.5309) centre (9.8684, 101.5215) ccw
  arc A7 (63.5351, 77.2224) -> (66.4388, 77.6061) centre (64.8079, 78.7694) ccw
  arc A8 (71.3254, 84.4568) -> (70.9598, 87.1692) centre (69.6971, 85.6182) ccw
  arc A9 (69.5236, 89.2106) -> (69.0767, 91.9424) centre (67.8754, 90.3434) ccw
  line L5 (0, 0) -> (41.1385, 99.317)
  arc A10 (71.651, 84.2245) -> (71.2123, 87.4794) centre (69.6971, 85.6182) ccw
  line L6 (71.651, 84.2245) -> (66.7645, 77.3738)
  arc A11 (63.2809, 76.9135) -> (66.7645, 77.3738) centre (64.8079, 78.7694) ccw
  arc A12 (63.2809, 76.9135) -> (9.6362, 99.1328) centre (0, 0) ccw
  arc A13 (7.5013, 101.9176) -> (9.6362, 99.1328) centre (9.8684, 101.5215) ccw
  line L7 (7.5013, 101.9176) -> (8.8908, 110.2206)
  arc A14 (11.5026, 112.212) -> (8.8908, 110.2206) centre (11.2579, 109.8245) ccw
  arc A15 (13.4679, 111.9931) -> (11.5026, 112.212) centre (0, 0) ccw
  line L8 (13.4679, 111.9931) -> (13.5275, 112.3149)
  arc A16 (16.2248, 114.2537) -> (13.5275, 112.3149) centre (15.8873, 111.8776) ccw
  arc A17 (69.317, 92.2622) -> (16.2248, 114.2537) centre (0, 0) ccw
  arc A18 (69.8533, 88.9841) -> (69.317, 92.2622) centre (67.8754, 90.3434) ccw
  line L9 (69.8533, 88.9841) -> (69.6679, 88.7143)
  arc A19 (71.2123, 87.4794) -> (69.6679, 88.7143) centre (0, 0) ccw
  point P0 (0, 0)
  point P1 (70.9598, 87.1692)
  point P2 (71.2123, 87.4794)
  dimension "d127" = 22.5
  constraints: 1 other
extrude "Extrusion9" cut sketch "Sketch6" against normal through all contours L1 A4 A8 L2 A7 A1 A6 L3 A0 A3 L4 A5 A2 A9 | L6 A11 A12 A13 L7 A14 A15 L8 A16 A17 A18 L9 A19 A10
pattern_circular "Circular Pattern1" count 8 over 360 about axis through (0, 0, -10) along (0, 0, 1) of "Extrusion9"
sketch "Block2" plane through (0, 0, 0) normal (0, 0, 1) x (1, 0, 0)
  line L0 (83.1381, 5.88) -> (71.258, 5.88)
  line L1 (71.258, 5.88) -> (71.258, -6)
  line L2 (71.258, -6) -> (83.1381, -6)
  line L3 (83.1381, -6) -> (83.1381, 5.88)
  line L4 (83.1381, 5.88) -> (71.258, -6) construction
  line L5 (71.258, 5.88) -> (83.1381, -6) construction
  circle A0 centre (77.198, -0.06) radius 2
  circle A1 centre (72.671, -4.587) radius 2.1
  circle A2 centre (81.725, -4.587) radius 2.1
  circle A3 centre (81.725, 4.467) radius 2.1
  circle A4 centre (72.671, 4.467) radius 2.1
  circle A5 centre (70.898, -0.06) radius 0.75
  line L6 (70.898, -0.06) -> (77.198, -0.06)
  dimension "d13" = 11.88
  dimension "d15" = 4.2
  dimension "d21" = 360
  dimension "d22" = 142.521
  dimension "d23" = 0
  dimension "d24" = 45
  dimension "d25" = 90
  dimension "d26" = 135
  dimension "d27" = 180
  dimension "d28" = -45
  dimension "d29" = 90
  dimension "d30" = 135
  dimension "d31" = 180
  dimension "d32" = -45
  dimension "d33" = 90
  dimension "d34" = 135
  dimension "d35" = 0
  dimension "d36" = -45
  dimension "d37" = 90
  dimension "d38" = 45
  dimension "d39" = 140.97
  dimension "d40" = 360
  dimension "d41" = 0
  dimension "d42" = -32.727
  dimension "d12" = 11.88
  dimension "d14" = 4
  dimension "d16" = 1.413
  dimension "d17" = 360
  dimension "d18" = 1.5
  dimension "d19" = 6.3
  constraints: 6 end point, 2 centre point, 2 coincident, 2 midpoint, 1 horizontal, 1 point on line, 21 other
  measures "d12" distance of L5.end L4.end
  measures "d14" diameter of A0
  measures "d18" diameter of A5
  measures "d19" distance of L6.end L6.start
body "Solid1"
